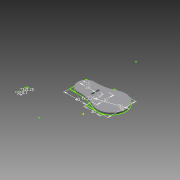
# Autodesk Inventor part: arm-servo
Saved by Autodesk Inventor 2013 (Build 170138000, 138)
## iProperties
Created: 2012-09-08
Part Number: arm-servo
Material: Generic
Document SubType Name: Modeling
Designer: frankenteddy
Density: 1 g/cm^3
Author: frankenteddy
Autodesk Inventor part; units mm, degrees
ref_plane "YZ Plane" through (0, 0, 0) normal (1, 0, 0) x (0, 1, 0)
ref_plane "XZ Plane" through (0, 0, 0) normal (0, 1, 0) x (-1, 0, 0)
ref_plane "XY Plane" through (0, 0, 0) normal (0, 0, 1) x (1, 0, 0)
sketch "Block1" plane through (0, 0, 0) normal (0, 0, 1) x (1, 0, 0)
  circle A0 centre (74.029, 24.2723) radius 1
  line L0 (49.279, 30.4723) -> (71.779, 30.4723)
  line L1 (71.779, 30.4723) -> (71.779, 18.0723)
  line L2 (71.779, 18.0723) -> (49.279, 18.0723)
  line L3 (49.279, 18.0723) -> (49.279, 30.4723)
  line L4 (49.279, 30.4723) -> (44.779, 30.4723)
  line L5 (44.779, 30.4723) -> (44.779, 18.0723)
  line L6 (44.779, 18.0723) -> (49.279, 18.0723)
  line L7 (49.279, 18.0723) -> (49.279, 30.4723)
  line L8 (71.779, 30.4723) -> (76.279, 30.4723)
  line L9 (76.279, 30.4723) -> (76.279, 18.0723)
  line L10 (76.279, 18.0723) -> (71.779, 18.0723)
  line L11 (71.779, 18.0723) -> (71.779, 30.4723)
  line L12 (44.779, 24.2723) -> (76.279, 24.2723) construction
  line L13 (47.029, 30.4723) -> (47.029, 18.0723) construction
  circle A1 centre (47.029, 24.2723) radius 1
  line L14 (74.029, 30.4723) -> (74.029, 18.0723) construction
  point P0 (60.979, 24.0984)
  dimension "d7" = 22.5
  dimension "d8" = 12.4
  dimension "d9" = 4.5
  dimension "d10" = 4.5
  dimension "d11" = 2
  dimension "d12" = 2
  measures "d7" distance of L1.end L2.end
  measures "d8" distance of L0.end L1.end
  measures "d9" distance of L6.end L5.end
  measures "d10" distance of L9.end L10.end
  measures "d11" diameter of A0
  measures "d12" diameter of A1
sketch "Sketch1" plane through (0, 0, 0) normal (0, 0, 1) x (1, 0, 0)
  line L0 (-92.7646, -8.503) -> (-89.7646, -8.503)
  line L1 (-89.7646, -8.503) -> (-89.7646, -11.753)
  line L2 (-89.7646, -11.753) -> (-92.7646, -11.753)
  line L3 (-92.7646, -11.753) -> (-92.7646, -8.503)
  line L4 (-92.7646, -21.6527) -> (-89.7646, -21.6527)
  line L5 (-89.7646, -21.6527) -> (-89.7646, -21.7527)
  line L6 (-89.7646, -21.7527) -> (-92.7646, -21.7527)
  line L7 (-92.7646, -21.7527) -> (-92.7646, -21.6527)
  line L8 (-51.3097, 56.2955) -> (-11.3097, 56.2955)
  line L9 (-11.3097, 56.2955) -> (-11.3097, 26.2955)
  line L10 (-11.3097, 26.2955) -> (-51.3097, 26.2955)
  line L11 (-51.3097, 26.2955) -> (-51.3097, 56.2955)
  line L12 (-51.3097, 41.2955) -> (-11.3097, 41.2955) construction
  line L13 (-21.3097, 48.2955) -> (-18.0597, 48.2955)
  line L14 (-18.0597, 48.2955) -> (-18.0597, 34.2955)
  line L15 (-18.0597, 34.2955) -> (-21.3097, 34.2955)
  line L16 (-21.3097, 34.2955) -> (-21.3097, 48.2955)
  line L17 (-21.3097, 41.2955) -> (-18.0597, 41.2955) construction
  line L18 (-11.3097, 66.2955) -> (18.6903, 66.2955)
  line L19 (18.6903, 66.2955) -> (18.6903, 16.2955)
  line L20 (18.6903, 16.2955) -> (-11.3097, 16.2955)
  line L21 (-11.3097, 16.2955) -> (-11.3097, 66.2955)
  line L22 (-11.3097, 41.2955) -> (18.6903, 41.2955) construction
  line L23 (-38.3097, 56.2955) -> (-38.3097, 26.2955) construction
  arc A0 (-38.3097, 56.2955) -> (-38.3097, 26.2955) centre (-36.1559, 41.2955) ccw
  circle A1 centre (9.1348, 41.2955) radius 25
  arc A2 (-31.9326, 56.2955) -> (-1.361, 63.9855) centre (-33.7351, 128.0749) ccw
  line L24 (-31.9326, 56.2955) -> (-31.9326, 53.1229)
  line L25 (-31.9326, 53.1229) -> (-1.361, 53.1229)
  line L26 (-1.361, 53.1229) -> (-1.361, 63.9855)
  arc A3 (-1.361, 18.6054) -> (-31.9326, 26.2955) centre (-33.7351, -45.4839) ccw
  line L27 (-31.9326, 26.2955) -> (-31.9326, 29.468)
  line L28 (-31.9326, 29.468) -> (-1.361, 29.468)
  line L29 (-1.361, 29.468) -> (-1.361, 18.6054)
  point P0 (0, 0)
  dimension "d0" = 3
  dimension "mat" = 3.25
  dimension "d2" = 3
  dimension "d3" = 0.1
  dimension "d23" = 40
  dimension "d24" = 30
  dimension "d29" = 3.25
  dimension "d30" = 14
  dimension "d31" = 30
  dimension "d38" = 30
  dimension "d39" = 50
  dimension "d42" = 13
  dimension "d43" = 50
  constraints: 60 end point, 12 parallel, 7 perpendicular, 7 point on circle, 6 midpoint, 5 horizontal, 5 symmetric about line, 4 centre point, 3 collinear, 3 point on line, 1 other
  measures "d0" distance of L1.end L3.start
  measures "mat" distance of L1.start L1.end
  measures "d2" distance of L5.end L7.start
  measures "d3" distance of L5.start L5.end
  measures "d23" distance of L9.end L10.end
  measures "d24" distance of L8.end L9.end
  measures "d29" distance of L14.end L15.end
  measures "d30" distance of L13.end L14.end
  measures "d31" distance between parallel lines of L11 L16
  measures "d38" distance of L19.end L20.end
  measures "d39" distance of L18.end L19.end
  measures "d42" distance between parallel lines of L23 L11
  measures "d43" diameter of A1
extrude "Extrusion6" add sketch "Sketch1" along normal blind 3.25 contours L8 L24 L25 A1 L28 L27 L10 A0 | L8 L9 A1 L25 L24 | L27 L28 A1 L9 L10 | A1 A2 L26 L25 L9 | L9 L25 A1 | A1 A2 | L25 L9 L28 A1 | L25 L26 A1 L19 L29 L28 L9 | L28 L9 A1 | L9 L28 L29 A3 A1 | A3 A1 | A1 L19
extrude "Extrusion7" add sketch "Sketch1" along normal blind 3.25 contours A2 L21 L8 | L8 L9 A1 L25 L24 | L21 A2 A1 L9 | A1 A2 L26 L25 L9 | L9 L25 A1
extrude "Extrusion8" add sketch "Sketch1" along normal blind 3.25 contours L27 L28 A1 L9 L10 | L10 L21 A3 | L9 A1 A3 L21 | L28 L9 A1 | L9 L28 L29 A3 A1
equation "\"d29\" = mat"
equation "\"d44\" = mat"
equation "\"d46\" = mat"
equation "\"d48\" = mat"
body "Solid6"
